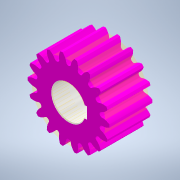
# Autodesk Inventor part: Pinion m10 Z18
Saved by Autodesk Inventor 2022 (Build 260153000, 153)
## iProperties
Created: 2022-01-08
Part Number: Pinion m10 Z18
Material: Generic
Document SubType Name: Modeling
Designer: Elia
Density: 1 g/cm^3
Appearance: Magenta
Author: Elia
Autodesk Inventor part; units mm, degrees
ref_plane "YZ Plane" through (0, 0, 0) normal (1, 0, 0) x (0, 1, 0)
ref_plane "XZ Plane" through (0, 0, 0) normal (0, 1, 0) x (-1, 0, 0)
ref_plane "XY Plane" through (0, 0, 0) normal (0, 0, 1) x (1, 0, 0)
sketch "Sketch1" plane through (0, 0, 0) normal (0, 0, 1) x (1, 0, 0)
  spline S0 degree 3 poles (-13.9983, 99.0154) (-13.6354, 98.5803) (-12.9095, 97.7102) (-11.8781, 96.3587) (-10.8923, 94.9739) (-9.9607, 93.5518) (-9.0883, 92.0926) (-8.2825, 90.5955) (-7.5538, 89.0594) (-6.9142, 87.4835) (-6.4818, 86.134) (-6.2049, 85.0339) (-6.0991, 84.1899) (-6.0007, 83.3463) (-5.8486, 82.5091) (-5.6194, 81.6902) (-5.3356, 80.8883) (-4.9597, 80.124) (-4.4911, 79.413) (-3.9271, 78.7728) (-3.3675, 78.3346) (-2.8885, 78.0312) (-2.5022, 77.8526) (-2.1066, 77.6957) (-1.6934, 77.5938) (-1.275, 77.5155) (-0.7079, 77.4906) (0, 77.5063) (0.7079, 77.4906) (1.275, 77.5155) (1.6934, 77.5938) (2.1066, 77.6957) (2.5022, 77.8526) (2.8885, 78.0312) (3.3675, 78.3346) (3.9271, 78.7728) (4.4911, 79.413) (4.9597, 80.124) (5.3356, 80.8883) (5.6194, 81.6902) (5.8486, 82.5091) (6.0007, 83.3463) (6.0991, 84.1899) (6.2049, 85.0339) (6.4818, 86.134) (6.9142, 87.4835) (7.5538, 89.0594) (8.2825, 90.5955) (9.0883, 92.0926) (9.9607, 93.5518) (10.8923, 94.9739) (11.8781, 96.3587) (12.9095, 97.7102) (13.6354, 98.5803) (13.9983, 99.0154) knots 0 0 0 0 0.169957 0.339916 0.509874 0.679831 0.849786 1.019738 1.189685 1.359624 1.52954 1.61451 1.699431 1.784405 1.869376 1.95433 2.039276 2.124226 2.209166 2.294083 2.378949 2.421442 2.463923 2.506416 2.548895 2.591387 2.633863 2.718846 2.803828 2.846304 2.888796 2.931276 2.973768 3.016249 3.058742 3.143608 3.228525 3.313466 3.398415 3.483361 3.568315 3.653287 3.73826 3.823181 3.908151 4.078068 4.248006 4.417953 4.587905 4.75786 4.927817 5.097775 5.267734 5.437691 5.437691 5.437691 5.437691
  circle A0 centre (0, 0) radius 77.5 construction
  circle A1 centre (0, 0) radius 84.5723 construction
  circle A2 centre (0, 0) radius 90
  circle A3 centre (0, 0) radius 100
  arc A4 (37.4438, 14.07) -> (37.4438, -14.07) centre (0, 0) ccw
  line L0 (37.4438, 14.07) -> (45.4, 14.07)
  line L1 (45.4, 14.07) -> (45.4, -14.07)
  line L2 (45.4, -14.07) -> (37.4438, -14.07)
  point P0 (-12.9191, 97.7025)
  point P1 (-11.8857, 96.3531)
  point P2 (-10.9013, 94.9677)
  point P3 (-9.9706, 93.5456)
  point P4 (-9.0994, 92.0863)
  point P5 (-8.2954, 90.589)
  point P6 (-7.5687, 89.0527)
  point P7 (-6.9343, 87.4762)
  point P8 (-6.4183, 85.8573)
  point P9 (-6.2219, 85.0306)
  point P10 (-6.1004, 84.1901)
  point P11 (-5.9918, 83.3473)
  point P12 (-5.8357, 82.5121)
  point P13 (-5.6103, 81.693)
  point P14 (-5.3203, 80.8946)
  point P15 (-4.9442, 80.1328)
  point P16 (-4.4751, 79.4247)
  point P17 (-3.9091, 78.7917)
  point P18 (-3.2454, 78.2629)
  point P19 (-2.884, 78.0393)
  point P20 (-2.5007, 77.8562)
  point P21 (-2.1036, 77.7049)
  point P22 (-1.6925, 77.5977)
  point P23 (-1.2738, 77.5254)
  point P24 (-0.8498, 77.4999)
  point P25 (0, 77.5)
  point P26 (0.8498, 77.4999)
  point P27 (1.2738, 77.5254)
  point P28 (1.6925, 77.5977)
  point P29 (2.1036, 77.7049)
  point P30 (2.5007, 77.8562)
  point P31 (2.884, 78.0393)
  point P32 (3.2454, 78.2629)
  point P33 (3.9091, 78.7917)
  point P34 (4.4751, 79.4247)
  point P35 (4.9442, 80.1328)
  point P36 (5.3203, 80.8946)
  point P37 (5.6103, 81.693)
  point P38 (5.8357, 82.5121)
  point P39 (5.9918, 83.3473)
  point P40 (6.1004, 84.1901)
  point P41 (6.2219, 85.0306)
  point P42 (6.4183, 85.8573)
  point P43 (6.9343, 87.4762)
  point P44 (7.5687, 89.0527)
  point P45 (8.2954, 90.589)
  point P46 (9.0994, 92.0863)
  point P47 (9.9706, 93.5456)
  point P48 (10.9013, 94.9677)
  point P49 (11.8857, 96.3531)
  point P50 (12.9191, 97.7025)
  point P51 (45.4, 0)
  dimension "d7" = 180
  dimension "d10" = 80
  dimension "d11" = 28.14
  dimension "d12" = 85.4
  constraints: 6 end point, 5 centre point, 4 point on circle, 2 perpendicular, 1 coincident, 1 horizontal, 1 horizontal alignment, 1 midpoint, 111 other
  measures "d7" diameter of A2
  measures "d10" diameter of A4
  measures "d11" distance of L0.end L1.end
extrude "Estrusione1" add sketch "Sketch1" against normal blind 105 contours A3 S0 A2 | S0 A2 A3 | A2 S0 | S0 A2 | L0 L1 L2 A4
extrude "Estrusione2" cut sketch "Sketch1" against normal blind 105 contours A3 S0 A2 | A2 S0 picked at (0.8724, 96.5809) picked at (-0.8263, 85.494)
pattern_circular "Serie circolare1" count 18 over 360 about axis through (0, 0, 0) along (0, 0, -1) of "Estrusione2"
surface extrude "SupEstrusione1" sketch "Sketch1" against normal blind 105 shown yes curves A2
surface extrude "SupEstrusione2" sketch "Sketch1" against normal blind 40 shown yes curves A4 L2 L1 L0
extrude "Estrusione3" cut sketch "Sketch1" against normal blind 105 contours L0 L1 L2 A4
chamfer "Smusso1" distance 2 angle 45 2 edges at (-40, 0, 0) (-40, 0, -105)
equation "\"Angolo_di_pressione\" = 20deg"
equation "\"Gioco_profilo_unità\" = 0.25"
equation "\"Raggio_circolare_unità\" = 0.35"
equation "\"Diametro_di_fondo\" = 155"
equation "\"Diametro_di_base\" = 169.14467"
equation "\"Angolo_elica\" = 0"
equation "\"Correzione_unità\" = 0"
equation "\"Modifica_aggiunta_unità\" = 0"
equation "\"Passo_circonferenziale\" = 31.415927"
equation "\"Spostamento_strumento_gioco\" = 0"
equation "\"Spostamento_strumento_totale\" = 0"
equation "\"Interno\" = 0"
